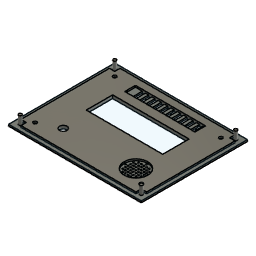
HousingLid v3 (Autodesk Fusion 360 design; units mm, degrees)
Autodesk Fusion 360 part; units mm, degrees
note: some values were not read from the file. Set by a fixed rule: which sketch regions a step uses; which face or edge a step refers to.
sketch "Sketch1" plane through (0, 0, 0) normal (0, 1, 0) x (1, 0, 0)
  line L0 (0, 0) -> (125, 0)
  line L1 (125, 0) -> (125, -100)
  line L2 (125, -100) -> (0, -100)
  line L3 (0, -100) -> (0, 0)
  dimension "d1" = 125
  dimension "d2" = 100
  constraint horizontal L0
  constraint vertical L1
  constraint horizontal L2
  constraint vertical L3
  constraint coincident L0.start L3.end
  measures "d1" distance of L0.start L0.end
  measures "d2" distance of L0.start L2.end
extrude "Extrude1" add sketch "Sketch1" along normal blind 2
sketch "Sketch2" plane through (0, 2, 0) normal (0, 1, 0) x (-1, 0, 0)
  line L0 (0, 100) -> (-125, 100)
  line L1 (-125, 100) -> (-125, 0)
  line L2 (-125, 0) -> (0, 0)
  line L3 (0, 0) -> (0, 100)
  line L4 (-10, 0) -> (-10, 3.3)
  line L5 (0, 3.3) -> (-3.3, 3.3)
  line L6 (-125, 100) -> (-121.7, 100)
  line L7 (-121.7, 100) -> (-121.7, 96.7)
  line L8 (-121.7, 96.7) -> (-125, 96.7)
  line L9 (-125, 96.7) -> (-125, 100)
  line L10 (-3.3, 3.3) -> (-121.7, 3.3)
  line L11 (-121.7, 3.3) -> (-121.7, 96.7)
  line L12 (-121.7, 96.7) -> (-3.3, 96.7)
  line L13 (-3.3, 96.7) -> (-3.3, 3.3)
  dimension "d5" = 3.3
  dimension "d6" = 3.3
  dimension "d7" = 3.3
  dimension "d8" = 3.3
  constraint coincident L2 L4.start
  constraint perpendicular L2 L4
  constraint coincident L3 L5.start
  constraint perpendicular L3 L5
  constraint horizontal L6
  constraint vertical L7
  constraint horizontal L8
  constraint vertical L9
  constraint coincident L0.end L1.start
  constraint horizontal L10
  constraint vertical L11
  constraint horizontal L12
  constraint vertical L13
  measures "d5" distance of L4.start L4.end
  measures "d6" distance of L5.start L5.end
  measures "d7" distance of L0.end L6.end
  measures "d8" distance of L0.end L8.end
extrude "Extrude2" add sketch "Sketch2" along normal blind 1 contours L10 L11 L12 L13
extrude "Extrude3" cut 1 faces at (42.7667, 2, 1.1) along direction (0, -1, 0) blind 0.5
sketch "Sketch3" plane through (0, 3, 0) normal (0, 1, 0) x (-1, 0, 0)
  line L0 (-3.3, 96.7) -> (-121.7, 96.7)
  line L1 (-121.7, 96.7) -> (-121.7, 3.3)
  line L2 (-121.7, 3.3) -> (-3.3, 3.3)
  line L3 (-3.3, 3.3) -> (-3.3, 96.7)
  line L4 (-3.3, 3.3) -> (-13.5, 3.3)
  line L5 (-13.5, 3.3) -> (-13.5, 13.5)
  line L6 (-13.5, 13.5) -> (-3.3, 13.5)
  line L7 (-3.3, 13.5) -> (-3.3, 3.3)
  line L8 (-3.3, 96.7) -> (-13.5, 96.7)
  line L9 (-13.5, 96.7) -> (-13.5, 86.5)
  line L10 (-13.5, 86.5) -> (-3.3, 86.5)
  line L11 (-3.3, 86.5) -> (-3.3, 96.7)
  line L12 (-121.7, 3.3) -> (-111.5, 3.3)
  line L13 (-111.5, 3.3) -> (-111.5, 13.5)
  line L14 (-111.5, 13.5) -> (-121.7, 13.5)
  line L15 (-121.7, 13.5) -> (-121.7, 3.3)
  line L16 (-121.7, 96.7) -> (-111.5, 96.7)
  line L17 (-111.5, 96.7) -> (-111.5, 86.5)
  line L18 (-111.5, 86.5) -> (-121.7, 86.5)
  line L19 (-121.7, 86.5) -> (-121.7, 96.7)
  dimension "d13" = 10.2
  dimension "d14" = 10.2
  dimension "d15" = 10.2
  dimension "d16" = 10.2
  dimension "d17" = 10.2
  dimension "d18" = 10.2
  dimension "d19" = 10.2
  dimension "d20" = 10.2
  constraint horizontal L4
  constraint vertical L5
  constraint horizontal L6
  constraint vertical L7
  constraint coincident L2.end L3.start
  constraint horizontal L8
  constraint vertical L9
  constraint horizontal L10
  constraint vertical L11
  constraint coincident L0.start L3.end
  constraint horizontal L12
  constraint vertical L13
  constraint horizontal L14
  constraint vertical L15
  constraint coincident L1.end L2.start
  constraint horizontal L16
  constraint vertical L17
  constraint horizontal L18
  constraint vertical L19
  constraint coincident L0.end L1.start
  measures "d13" distance of L2.end L4.end
  measures "d14" distance of L2.end L6.end
  measures "d15" distance of L0.start L8.end
  measures "d16" distance of L0.start L10.end
  measures "d17" distance of L1.end L12.end
  measures "d18" distance of L1.end L14.end
  measures "d19" distance of L0.end L16.end
  measures "d20" distance of L0.end L18.end
extrude "Extrude4" cut sketch "Sketch3" against normal blind 1 contours L0 L3 L8 L9 L10 L11 | L0 L1 L16 L17 L18 L19 | L2 L3 L4 L5 L6 L7 | L1 L2 L12 L13 L14 L15
extrude "Extrude5" cut 4 faces at (6.7, 2, 6.7) (118.3, 2, 6.7) (118.3, 2, 93.3) (6.7, 2, 93.3) along direction (0, -1, 0) blind 0.5
sketch "Sketch4" plane through (0, 1.5, 0) normal (0, 1, 0) x (-1, 0, 0)
  line L0 (-3.3, 13.5) -> (-13.5, 13.5)
  line L1 (-13.5, 13.5) -> (-13.5, 3.3)
  line L2 (-13.5, 3.3) -> (-111.5, 3.3)
  line L3 (-111.5, 3.3) -> (-111.5, 13.5)
  line L4 (-111.5, 13.5) -> (-121.7, 13.5)
  line L5 (-121.7, 13.5) -> (-121.7, 86.5)
  line L6 (-121.7, 86.5) -> (-111.5, 86.5)
  line L7 (-111.5, 86.5) -> (-111.5, 96.7)
  line L8 (-111.5, 96.7) -> (-13.5, 96.7)
  line L9 (-13.5, 96.7) -> (-13.5, 86.5)
  line L10 (-13.5, 86.5) -> (-3.3, 86.5)
  line L11 (-3.3, 86.5) -> (-3.3, 13.5)
  line L12 (0, 100) -> (-125, 100)
  line L13 (-125, 100) -> (-125, 0)
  line L14 (-125, 0) -> (0, 0)
  line L15 (0, 0) -> (0, 100)
  line L16 (0, 0) -> (-8, 0)
  line L17 (0, 8) -> (0, 0)
  circle A0 centre (-8, 8) radius 1.5
  line L18 (0, 100) -> (-8, 100)
  line L19 (-8, 100) -> (-8, 92)
  line L20 (-8, 92) -> (0, 92)
  line L21 (0, 92) -> (0, 100)
  circle A1 centre (-8, 92) radius 1.5
  line L22 (-125, 100) -> (-117, 100)
  line L23 (-117, 100) -> (-117, 92)
  line L24 (-117, 92) -> (-125, 92)
  line L25 (-125, 92) -> (-125, 100)
  circle A2 centre (-117, 92) radius 1.5
  line L26 (-125, 0) -> (-117, 0)
  line L27 (-117, 0) -> (-117, 8)
  line L28 (-117, 8) -> (-125, 8)
  line L29 (-125, 8) -> (-125, 0)
  circle A3 centre (-117, 8) radius 1.5
  dimension "d25" = 8
  dimension "d26" = 8
  dimension "d27" = 3
  dimension "d28" = 8
  dimension "d29" = 8
  dimension "d30" = 3
  dimension "d31" = 3
  dimension "d32" = 3
  constraint horizontal L16
  constraint vertical L17
  constraint coincident L14.end L15.start
  constraint horizontal L18
  constraint vertical L19
  constraint horizontal L20
  constraint vertical L21
  constraint coincident L12.start L15.end
  constraint coincident L19.end L20.start
  constraint horizontal L22
  constraint vertical L23
  constraint horizontal L24
  constraint vertical L25
  constraint coincident L12.end L13.start
  constraint coincident L23.end L24.start
  constraint horizontal L26
  constraint vertical L27
  constraint horizontal L28
  constraint vertical L29
  constraint coincident L13.end L14.start
  constraint coincident L27.end L28.start
  measures "d25" distance of L14.end L16.end
  measures "d26" distance of L14.end L17.start
  measures "d27" diameter of A0
  measures "d28" distance of L12.start L18.end
  measures "d29" distance of L12.start L20.end
  measures "d30" diameter of A1
  measures "d31" diameter of A2
  measures "d32" diameter of A3
extrude "Extrude6" add sketch "Sketch4" along normal blind 5 contours L19 L20 A1 | L19 L20 A1 | L23 L24 A2 | L23 L24 A2 | L27 L28 A3 | L27 L28 A3 | A0
extrude "Extrude7" add 4 faces at (8.1827, 6.5, 8.5095) (8.0374, 6.5, 90.9381) (117.5343, 6.5, 7.6091) (116.9626, 6.5, 92.2038) along direction (0, 1, 0) blind 8
extrude "Extrude8" cut 4 faces at (8.1827, 14.5, 8.5095) (8.0374, 14.5, 90.9381) (117.5343, 14.5, 7.6091) (116.9626, 14.5, 92.2038) along direction (0, -1, 0) blind 14.5
sketch "Sketch5" plane through (0, 1.5, 0) normal (0, 1, 0) x (-1, 0, 0)
  circle A0 centre (-8, 8) radius 1.5
  circle A1 centre (-117, 8) radius 1.5
  circle A2 centre (-8, 92) radius 1.5
  circle A3 centre (-117, 92) radius 1.5
  line L0 (-3.3, 13.5) -> (-13.5, 13.5)
  line L1 (-13.5, 13.5) -> (-13.5, 3.3)
  line L2 (-13.5, 3.3) -> (-111.5, 3.3)
  line L3 (-111.5, 3.3) -> (-111.5, 13.5)
  line L4 (-111.5, 13.5) -> (-121.7, 13.5)
  line L5 (-121.7, 13.5) -> (-121.7, 86.5)
  line L6 (-121.7, 86.5) -> (-111.5, 86.5)
  line L7 (-111.5, 86.5) -> (-111.5, 96.7)
  line L8 (-111.5, 96.7) -> (-13.5, 96.7)
  line L9 (-13.5, 96.7) -> (-13.5, 86.5)
  line L10 (-13.5, 86.5) -> (-3.3, 86.5)
  line L11 (-3.3, 86.5) -> (-3.3, 13.5)
  line L12 (0, 100) -> (-125, 100)
  line L13 (-125, 100) -> (-125, 0)
  line L14 (-125, 0) -> (0, 0)
  line L15 (0, 0) -> (0, 100)
  circle A4 centre (-8, 8) radius 1.65
  circle A5 centre (-8, 92) radius 1.65
  circle A6 centre (-117, 92) radius 1.65
  circle A7 centre (-117, 8) radius 1.65
  dimension "d39" = 3.3
  dimension "d40" = 3.3
  dimension "d41" = 3.3
  dimension "d42" = 3.3
  constraint concentric A0 A4
  constraint concentric A2 A5
  constraint concentric A3 A6
  constraint concentric A1 A7
  measures "d39" diameter of A4
  measures "d40" diameter of A5
  measures "d41" diameter of A6
  measures "d42" diameter of A7
extrude "Extrude9" cut sketch "Sketch5" against normal blind 1.5 contours A4 | A5 | A6 | A7
delete_face "DeleteFace1" 1 faces at (6.3521, 0.5, 7.9178)
delete_face "DeleteFace2" 1 faces at (9.4491, 0.5, 91.2109)
delete_face "DeleteFace3" 1 faces at (117.7527, 0.5, 93.4683)
delete_face "DeleteFace4" 1 faces at (117.7527, 0.5, 9.4683)
sketch "Sketch6" plane through (0, 0, 0) normal (0, -1, 0) x (1, 0, 0)
  line L0 (125, 100) -> (0, 100)
  line L1 (0, 100) -> (0, 0)
  line L2 (0, 0) -> (125, 0)
  line L3 (125, 0) -> (125, 100)
  line L4 (0, 0) -> (3, 0)
  line L5 (0, 3) -> (0, 0)
  line L6 (0, 100) -> (3, 100)
  line L7 (0, 97) -> (0, 100)
  line L8 (125, 100) -> (122, 100)
  line L9 (125, 97) -> (125, 100)
  line L10 (125, 0) -> (122, 0)
  line L11 (125, 3) -> (125, 0)
  circle A0 centre (122, 3) radius 1.65
  circle A1 centre (3, 3) radius 1.65
  circle A2 centre (3, 97) radius 1.65
  circle A3 centre (122, 97) radius 1.65
  dimension "d45" = 3
  dimension "d46" = 3
  dimension "d47" = 3
  dimension "d48" = 3
  dimension "d49" = 3
  dimension "d50" = 3.3
  dimension "d51" = 3.3
  dimension "d52" = 3.3
  dimension "d53" = 3.3
  constraint horizontal L4
  constraint vertical L5
  constraint coincident L1.end L2.start
  constraint horizontal L6
  constraint vertical L7
  constraint coincident L0.end L1.start
  constraint horizontal L8
  constraint vertical L9
  constraint coincident L0.start L3.end
  constraint horizontal L10
  constraint vertical L11
  constraint coincident L2.end L3.start
  measures "d45" distance of L0.end L7.start
  measures "d46" distance of L0.start L8.end
  measures "d47" distance of L0.start L9.start
  measures "d48" distance of L2.end L10.end
  measures "d49" distance of L2.end L11.start
  measures "d50" diameter of A0
  measures "d51" diameter of A1
  measures "d52" diameter of A2
  measures "d53" diameter of A3
extrude "Extrude10" cut sketch "Sketch6" against normal blind 1.5 contours A0 | A1 | A2 | A3
sketch "Sketch7" plane through (0, 1.5, 0) normal (0, 1, 0) x (-1, 0, 0)
  circle A0 centre (-3, 3) radius 1.65
  circle A1 centre (-122, 3) radius 1.65
  circle A2 centre (-3, 97) radius 1.65
  circle A3 centre (-122, 97) radius 1.65
  line L0 (-3.3, 13.5) -> (-13.5, 13.5)
  line L1 (-13.5, 13.5) -> (-13.5, 3.3)
  line L2 (-13.5, 3.3) -> (-111.5, 3.3)
  line L3 (-111.5, 3.3) -> (-111.5, 13.5)
  line L4 (-111.5, 13.5) -> (-121.7, 13.5)
  line L5 (-121.7, 13.5) -> (-121.7, 86.5)
  line L6 (-121.7, 86.5) -> (-111.5, 86.5)
  line L7 (-111.5, 86.5) -> (-111.5, 96.7)
  line L8 (-111.5, 96.7) -> (-13.5, 96.7)
  line L9 (-13.5, 96.7) -> (-13.5, 86.5)
  line L10 (-13.5, 86.5) -> (-3.3, 86.5)
  line L11 (-3.3, 86.5) -> (-3.3, 13.5)
  line L12 (0, 100) -> (-125, 100)
  line L13 (-125, 100) -> (-125, 0)
  line L14 (-125, 0) -> (0, 0)
  line L15 (0, 0) -> (0, 100)
  line L16 (0, 0) -> (-8.3, 0)
  line L17 (-8.3, 0) -> (-8.3, 8.3)
  line L18 (-8.3, 8.3) -> (0, 8.3)
  line L19 (0, 8.3) -> (0, 0)
  line L20 (-3.3, 13.5) -> (-3.3, 8.3)
  line L21 (-13.5, 3.3) -> (-8.3, 3.3)
  line L22 (-111.5, 3.3) -> (-116.7, 3.3)
  line L23 (-121.7, 13.5) -> (-121.7, 8.3)
  line L24 (-125, 0) -> (-116.7, 0)
  line L25 (-116.7, 0) -> (-116.7, 8.3)
  line L26 (-116.7, 8.3) -> (-125, 8.3)
  line L27 (-125, 8.3) -> (-125, 0)
  line L28 (-3.3, 86.5) -> (-13.5, 86.5)
  line L29 (-13.5, 86.5) -> (-13.5, 91.7)
  line L30 (-13.5, 91.7) -> (-3.3, 91.7)
  line L31 (-3.3, 91.7) -> (-3.3, 86.5)
  line L32 (-13.5, 96.7) -> (-8.3, 96.7)
  line L33 (-8.3, 96.7) -> (-8.3, 91.7)
  line L34 (-13.5, 91.7) -> (-13.5, 96.7)
  line L35 (-111.5, 96.7) -> (-116.7, 96.7)
  line L36 (-116.7, 96.7) -> (-116.7, 86.5)
  line L37 (-116.7, 86.5) -> (-111.5, 86.5)
  line L38 (-111.5, 86.5) -> (-111.5, 96.7)
  line L39 (-121.7, 86.5) -> (-111.5, 86.5)
  line L40 (-111.5, 86.5) -> (-111.5, 91.7)
  line L41 (-111.5, 91.7) -> (-121.7, 91.7)
  line L42 (-121.7, 91.7) -> (-121.7, 86.5)
  dimension "d59" = 8.3
  dimension "d60" = 8.3
  dimension "d61" = 5.2
  dimension "d62" = 5.2
  dimension "d63" = 8.3
  dimension "d64" = 8.3
  dimension "d65" = 5.2
  dimension "d66" = 5.2
  dimension "d67" = 5.2
  dimension "d68" = 5.2
  constraint horizontal L16
  constraint vertical L17
  constraint horizontal L18
  constraint vertical L19
  constraint coincident L14.end L15.start
  constraint coincident L0.start L11.end
  constraint coincident L18 L20.end
  constraint perpendicular L18 L20
  constraint coincident L1.end L2.start
  constraint coincident L17 L21.end
  constraint perpendicular L17 L21
  constraint coincident L2.end L3.start
  constraint perpendicular L3 L22
  constraint coincident L4.end L5.start
  constraint perpendicular L4 L23
  constraint horizontal L24
  constraint vertical L25
  constraint horizontal L26
  constraint vertical L27
  constraint coincident L13.end L14.start
  constraint horizontal L28
  constraint vertical L29
  constraint horizontal L30
  constraint vertical L31
  constraint coincident L10.end L11.start
  constraint horizontal L32
  constraint vertical L33
  constraint vertical L34
  constraint coincident L8.end L9.start
  constraint horizontal L35
  constraint vertical L36
  constraint horizontal L37
  constraint vertical L38
  constraint coincident L6 L36.end
  constraint coincident L7.end L8.start
  constraint horizontal L39
  constraint vertical L40
  constraint horizontal L41
  constraint vertical L42
  constraint coincident L5.end L6.start
  measures "d59" distance of L14.end L16.end
  measures "d60" distance of L14.end L18.end
  measures "d61" distance of L2.end L22.end
  measures "d62" distance of L4.end L23.end
  measures "d63" distance of L13.end L24.end
  measures "d64" distance of L13.end L26.end
  measures "d65" distance of L10.end L30.end
  measures "d66" distance of L8.end L32.end
  measures "d67" distance of L7.end L35.end
  measures "d68" distance of L5.end L41.end
extrude "Extrude11" add sketch "Sketch7" along normal blind 1.5 contours L0 L1 L17 L18 L20 L21 | L9 L10 L28 L29 L30 L31 | L3 L4 L22 L23 L25 L26 | L9 L30 L32 L33 L34 | L7 L35 L36 L38 L41 | L6 L36 L39 L41 L42 | L6 L7 L36 L37 L38 L39 L40 L41
delete_face "DeleteFace5" 1 faces at (121.2473, 1, 1.5317)
sketch "Sketch8" plane through (0, 1.5, 0) normal (0, 1, 0) x (-1, 0, 0)
  line L0 (-116.7, 96.7) -> (-8.3, 96.7)
  line L1 (-8.3, 96.7) -> (-8.3, 91.7)
  line L2 (-8.3, 91.7) -> (-3.3, 91.7)
  line L3 (-3.3, 91.7) -> (-3.3, 8.3)
  line L4 (-3.3, 8.3) -> (-8.3, 8.3)
  line L5 (-8.3, 8.3) -> (-8.3, 3.3)
  line L6 (-8.3, 3.3) -> (-116.7, 3.3)
  line L7 (-116.7, 3.3) -> (-116.7, 8.3)
  line L8 (-116.7, 8.3) -> (-121.7, 8.3)
  line L9 (-121.7, 8.3) -> (-121.7, 91.7)
  line L10 (-121.7, 91.7) -> (-116.7, 91.7)
  line L11 (-116.7, 91.7) -> (-116.7, 96.7)
  line L12 (0, 100) -> (-125, 100)
  line L13 (-125, 100) -> (-125, 0)
  line L14 (-125, 0) -> (0, 0)
  line L15 (0, 0) -> (0, 100)
delete_face "DeleteFace6" 1 faces at (4.4079, 1, 97.8604)
delete_face "DeleteFace7" 1 faces at (4.6479, 1, 2.9178)
delete_face "DeleteFace8" 1 faces at (122.4469, 1, 98.5883)
sketch "Sketch9" plane through (0, 1.5, 0) normal (0, 1, 0) x (-1, 0, 0)
  line L0 (0, 0) -> (-5.5, 0)
  line L1 (0, 5.5) -> (0, 0)
  line L2 (0, 100) -> (-5, 100)
  line L3 (0, 95) -> (0, 100)
  line L4 (-125, 100) -> (-119.5, 100)
  line L5 (-125, 94.5) -> (-125, 100)
  line L6 (0, 100) -> (-5.5, 100)
  line L7 (0, 94.5) -> (0, 100)
  line L8 (-125, 0) -> (-119.5, 0)
  line L9 (-125, 5.5) -> (-125, 0)
  circle A0 centre (-119.5, 5.5) radius 1.5
  circle A1 centre (-119.5, 94.5) radius 1.5
  circle A2 centre (-5.5, 94.5) radius 1.5
  circle A3 centre (-5.5, 5.5) radius 1.5
  dimension "d71" = 5.5
  dimension "d72" = 5.5
  dimension "d73" = 5.5
  dimension "d74" = 5.5
  dimension "d75" = 5.5
  dimension "d76" = 5.5
  dimension "d77" = 3
  dimension "d78" = 3
  dimension "d79" = 3
  dimension "d80" = 3
  constraint horizontal L0
  constraint vertical L1
  constraint coincident L0.start L1.end
  constraint horizontal L2
  constraint vertical L3
  constraint horizontal L4
  constraint vertical L5
  constraint horizontal L6
  constraint vertical L7
  constraint horizontal L8
  constraint vertical L9
  measures "d71" distance of L0.start L0.end
  measures "d72" distance of L0.start L1.start
  measures "d73" distance of L4.start L4.end
  measures "d74" distance of L4.start L5.start
  measures "d75" distance of L8.start L8.end
  measures "d76" distance of L8.start L9.start
  measures "d77" diameter of A0
  measures "d78" diameter of A1
  measures "d79" diameter of A2
  measures "d80" diameter of A3
extrude "Extrude12" add sketch "Sketch9" along normal blind 8
sketch "Sketch10" plane through (0, 3, 0) normal (0, 1, 0) x (-1, 0, 0)
  line L0 (-116.7, 3.3) -> (-8.3, 3.3)
  line L1 (-8.3, 3.3) -> (-8.3, 8.3)
  line L2 (-8.3, 8.3) -> (-3.3, 8.3)
  line L3 (-3.3, 8.3) -> (-3.3, 91.7)
  line L4 (-3.3, 91.7) -> (-8.3, 91.7)
  line L5 (-8.3, 91.7) -> (-8.3, 96.7)
  line L6 (-8.3, 96.7) -> (-116.7, 96.7)
  line L7 (-116.7, 96.7) -> (-116.7, 91.7)
  line L8 (-116.7, 91.7) -> (-121.7, 91.7)
  line L9 (-121.7, 91.7) -> (-121.7, 8.3)
  line L10 (-121.7, 8.3) -> (-116.7, 8.3)
  line L11 (-116.7, 8.3) -> (-116.7, 3.3)
  line L12 (-12.5, 12.5) -> (-12.5, 0)
  line L13 (0, 0) -> (-7.5, 0)
  line L14 (-7.5, 0) -> (-7.5, 7.5)
  line L15 (-7.5, 7.5) -> (-117.5, 7.5)
  line L16 (-117.5, 7.5) -> (-117.5, 92.5)
  line L17 (-117.5, 92.5) -> (-7.5, 92.5)
  line L18 (-7.5, 92.5) -> (-7.5, 7.5)
  line L19 (-26.5, 28.5) -> (-98.5, 28.5)
  line L20 (-98.5, 28.5) -> (-98.5, 53.3)
  line L21 (-98.5, 53.3) -> (-26.5, 53.3)
  line L22 (-26.5, 53.3) -> (-26.5, 28.5)
  line L23 (-117.5, 92.5) -> (-117.5, 79)
  line L24 (-117.5, 92.5) -> (-94.5, 92.5)
  line L25 (-117.5, 79) -> (-117.5, 92.5)
  circle A0 centre (-94.5, 79) radius 3.5
  line L26 (-7.5, 92.5) -> (-27.5, 92.5)
  line L27 (-7.5, 77.5) -> (-7.5, 92.5)
  circle A1 centre (-27.5, 77.5) radius 9
  line L28 (-7.5, 7.5) -> (-29.5, 7.5)
  line L29 (-29.5, 7.5) -> (-29.5, 10)
  line L30 (-29.5, 10) -> (-95.5, 10)
  line L31 (-95.5, 10) -> (-95.5, 20)
  line L32 (-95.5, 20) -> (-29.5, 20)
  line L33 (-29.5, 20) -> (-29.5, 10)
  line L34 (-33, 10) -> (-36, 10)
  line L35 (-36, 10) -> (-36, 20)
  line L36 (-36, 20) -> (-33, 20)
  line L37 (-33, 20) -> (-33, 10)
  line L38 (-39, 20) -> (-42, 20)
  line L39 (-42, 20) -> (-42, 10)
  line L40 (-42, 10) -> (-39, 10)
  line L41 (-39, 10) -> (-39, 20)
  line L42 (-45, 10) -> (-48, 10)
  line L43 (-48, 10) -> (-48, 20)
  line L44 (-48, 20) -> (-45, 20)
  line L45 (-45, 20) -> (-45, 10)
  line L46 (-51, 20) -> (-54, 20)
  line L47 (-54, 20) -> (-54, 10)
  line L48 (-54, 10) -> (-51, 10)
  line L49 (-51, 10) -> (-51, 20)
  line L50 (-57, 10) -> (-60, 10)
  line L51 (-60, 10) -> (-60, 20)
  line L52 (-60, 20) -> (-57, 20)
  line L53 (-57, 20) -> (-57, 10)
  line L54 (-63, 20) -> (-66, 20)
  line L55 (-66, 20) -> (-66, 10)
  line L56 (-66, 10) -> (-63, 10)
  line L57 (-63, 10) -> (-63, 20)
  line L58 (-69, 10) -> (-72, 10)
  line L59 (-72, 10) -> (-72, 20)
  line L60 (-72, 20) -> (-69, 20)
  line L61 (-69, 20) -> (-69, 10)
  line L62 (-75, 10) -> (-78, 10)
  line L63 (-78, 10) -> (-78, 20)
  line L64 (-78, 20) -> (-75, 20)
  line L65 (-75, 20) -> (-75, 10)
  line L66 (-81, 10) -> (-84, 10)
  line L67 (-84, 10) -> (-84, 20)
  line L68 (-84, 20) -> (-81, 20)
  line L69 (-81, 20) -> (-81, 10)
  line L70 (-87, 10) -> (-90, 10)
  line L71 (-90, 10) -> (-90, 20)
  line L72 (-90, 20) -> (-87, 20)
  line L73 (-87, 20) -> (-87, 10)
  line L74 (-93, 10) -> (-95.5, 10)
  line L75 (-95.5, 10) -> (-95.5, 20)
  line L76 (-95.5, 20) -> (-93, 20)
  line L77 (-93, 20) -> (-93, 10)
  dimension "d85" = 7.5
  dimension "d86" = 7.5
  dimension "d87" = 110
  dimension "d88" = 85
  dimension "d92" = 24.8
  dimension "d93" = 23
  dimension "d94" = 13.5
  dimension "d95" = 7
  dimension "d96" = 20
  dimension "d97" = 15
  dimension "d98" = 18
  dimension "d99" = 22
  dimension "d100" = 66
  dimension "d101" = 10
  constraint coincident L13.start origin
  constraint horizontal L13
  constraint perpendicular L13 L14
  constraint horizontal L15
  constraint vertical L16
  constraint horizontal L17
  constraint vertical L18
  constraint horizontal L19
  constraint vertical L20
  constraint horizontal L21
  constraint vertical L22
  constraint coincident L16 L23.end
  constraint horizontal L24
  constraint vertical L25
  constraint horizontal L26
  constraint vertical L27
  constraint perpendicular L1 L28
  constraint perpendicular L15 L29
  constraint horizontal L30
  constraint vertical L31
  constraint horizontal L32
  constraint vertical L33
  constraint horizontal L34
  constraint vertical L35
  constraint horizontal L36
  constraint vertical L37
  constraint coincident L32 L35.end
  constraint coincident L30 L34.start
  constraint horizontal L38
  constraint vertical L39
  constraint horizontal L40
  constraint vertical L41
  constraint coincident L30 L39.end
  constraint coincident L32 L38.start
  constraint horizontal L42
  constraint vertical L43
  constraint horizontal L44
  constraint vertical L45
  constraint coincident L32 L43.end
  constraint coincident L30 L42.start
  constraint horizontal L46
  constraint vertical L47
  constraint horizontal L48
  constraint vertical L49
  constraint coincident L30 L47.end
  constraint coincident L32 L46.start
  constraint horizontal L50
  constraint vertical L51
  constraint horizontal L52
  constraint vertical L53
  constraint coincident L32 L51.end
  constraint coincident L30 L50.start
  constraint horizontal L54
  constraint vertical L55
  constraint horizontal L56
  constraint vertical L57
  constraint coincident L30 L55.end
  constraint coincident L32 L54.start
  constraint horizontal L58
  constraint vertical L59
  constraint horizontal L60
  constraint vertical L61
  constraint coincident L32 L59.end
  constraint coincident L30 L58.start
  constraint horizontal L62
  constraint vertical L63
  constraint horizontal L64
  constraint vertical L65
  constraint coincident L32 L63.end
  constraint coincident L30 L62.start
  constraint horizontal L66
  constraint vertical L67
  constraint horizontal L68
  constraint vertical L69
  constraint coincident L32 L67.end
  constraint coincident L30 L66.start
  constraint horizontal L70
  constraint vertical L71
  constraint horizontal L72
  constraint vertical L73
  constraint coincident L32 L71.end
  constraint coincident L30 L70.start
  constraint horizontal L74
  constraint vertical L75
  constraint horizontal L76
  constraint vertical L77
  constraint coincident L30 L74.start
  measures "d85" distance of L13.start L13.end
  measures "d86" distance of L13.end L14.end
  measures "d87" distance of L14.end L15.end
  measures "d88" distance of L14.end L17.end
  measures "d92" distance of L19.start L21.end
  measures "d93" distance of L16.end L24.end
  measures "d94" distance of L16.end L23.end
  measures "d95" diameter of A0
  measures "d96" distance of L17.end L26.end
  measures "d97" distance of L17.end L27.start
  measures "d98" diameter of A1
  measures "d99" distance of L14.end L28.end
  measures "d100" distance of L29.end L30.end
  measures "d101" distance of L29.end L32.end
extrude "Extrude13" cut sketch "Sketch10" against normal blind 3 contours L19 L20 L21 L22 | A0 | L30 L32 L35 L41 | L30 L32 L39 L45 | L30 L32 L43 L49 | L30 L32 L47 L53 | L30 L32 L51 L57 | L30 L32 L55 L61 | L30 L32 L59 L65 | L30 L32 L63 L69 | L30 L32 L67 L73 | L30 L32 L71 L77
delete_face "DeleteFace9" 1 faces at (91.0044, 1, 78.8255)
sketch "Sketch11" plane through (0, 3, 0) normal (0, 1, 0) x (-1, 0, 0)
  line L0 (-87, 20) -> (-84, 20)
  line L1 (-84, 20) -> (-84, 10)
  line L2 (-84, 10) -> (-87, 10)
  line L3 (-87, 10) -> (-87, 20)
  line L4 (-63, 20) -> (-60, 20)
  line L5 (-60, 20) -> (-60, 10)
  line L6 (-60, 10) -> (-63, 10)
  line L7 (-63, 10) -> (-63, 20)
  line L8 (-39, 20) -> (-36, 20)
  line L9 (-36, 20) -> (-36, 10)
  line L10 (-36, 10) -> (-39, 10)
  line L11 (-39, 10) -> (-39, 20)
  line L12 (-45, 10) -> (-45, 20)
  line L13 (-45, 20) -> (-42, 20)
  line L14 (-42, 20) -> (-42, 10)
  line L15 (-42, 10) -> (-45, 10)
  line L16 (-69, 10) -> (-69, 20)
  line L17 (-69, 20) -> (-66, 20)
  line L18 (-66, 20) -> (-66, 10)
  line L19 (-66, 10) -> (-69, 10)
  line L20 (-93, 20) -> (-90, 20)
  line L21 (-90, 20) -> (-90, 10)
  line L22 (-90, 10) -> (-93, 10)
  line L23 (-93, 10) -> (-93, 20)
  line L24 (-81, 20) -> (-78, 20)
  line L25 (-78, 20) -> (-78, 10)
  line L26 (-78, 10) -> (-81, 10)
  line L27 (-81, 10) -> (-81, 20)
  line L28 (-57, 10) -> (-57, 20)
  line L29 (-57, 20) -> (-54, 20)
  line L30 (-54, 20) -> (-54, 10)
  line L31 (-54, 10) -> (-57, 10)
  line L32 (-98.5, 28.5) -> (-98.5, 53.3)
  line L33 (-98.5, 53.3) -> (-26.5, 53.3)
  line L34 (-26.5, 53.3) -> (-26.5, 28.5)
  line L35 (-26.5, 28.5) -> (-98.5, 28.5)
  line L36 (-51, 20) -> (-48, 20)
  line L37 (-48, 20) -> (-48, 10)
  line L38 (-48, 10) -> (-51, 10)
  line L39 (-51, 10) -> (-51, 20)
  line L40 (-75, 20) -> (-72, 20)
  line L41 (-72, 20) -> (-72, 10)
  line L42 (-72, 10) -> (-75, 10)
  line L43 (-75, 10) -> (-75, 20)
  line L44 (-116.7, 3.3) -> (-8.3, 3.3)
  line L45 (-8.3, 3.3) -> (-8.3, 8.3)
  line L46 (-8.3, 8.3) -> (-3.3, 8.3)
  line L47 (-3.3, 8.3) -> (-3.3, 91.7)
  line L48 (-3.3, 91.7) -> (-8.3, 91.7)
  line L49 (-8.3, 91.7) -> (-8.3, 96.7)
  line L50 (-8.3, 96.7) -> (-116.7, 96.7)
  line L51 (-116.7, 96.7) -> (-116.7, 91.7)
  line L52 (-116.7, 91.7) -> (-121.7, 91.7)
  line L53 (-121.7, 91.7) -> (-121.7, 8.3)
  line L54 (-121.7, 8.3) -> (-116.7, 8.3)
  line L55 (-116.7, 8.3) -> (-116.7, 3.3)
  line L56 (-37.5, 10) -> (-37.5, 7.5)
  line L57 (-37.5, 7.5) -> (0, 7.5)
  line L58 (0, 0) -> (-7.5, 0)
  line L59 (-7.5, 0) -> (-7.5, 7.5)
  line L60 (-7.5, 7.5) -> (0, 7.5)
  line L61 (0, 7.5) -> (0, 0)
  line L62 (-125, 100) -> (-117.5, 100)
  line L63 (-117.5, 100) -> (-117.5, 92.5)
  line L64 (-117.5, 92.5) -> (-125, 92.5)
  line L65 (-125, 92.5) -> (-125, 100)
  line L66 (-7.5, 7.5) -> (-117.5, 7.5)
  line L67 (-117.5, 7.5) -> (-117.5, 92.5)
  line L68 (-117.5, 92.5) -> (-7.5, 92.5)
  line L69 (-7.5, 92.5) -> (-7.5, 7.5)
  line L70 (-117.5, 7.5) -> (-95.5, 7.5)
  line L71 (-95.5, 7.5) -> (-95.5, 10)
  line L72 (-7.5, 7.5) -> (-29.5, 7.5)
  line L73 (-29.5, 7.5) -> (-29.5, 10)
  line L74 (-29.5, 10) -> (-95.5, 10)
  line L75 (-95.5, 10) -> (-95.5, 20)
  line L76 (-95.5, 20) -> (-29.5, 20)
  line L77 (-29.5, 20) -> (-29.5, 10)
  line L78 (-117.5, 92.5) -> (-97.5, 92.5)
  line L79 (-97.5, 92.5) -> (-97.5, 77.5)
  line L80 (-97.5, 77.5) -> (-117.5, 77.5)
  line L81 (-117.5, 77.5) -> (-117.5, 92.5)
  circle A0 centre (-97.5, 77.5) radius 11.1
  dimension "d104" = 2.5
  dimension "d105" = 7.5
  dimension "d106" = 7.5
  dimension "d107" = 7.5
  dimension "d108" = 22
  dimension "d109" = 22
  dimension "d110" = 20
  dimension "d111" = 15
  dimension "d112" = 22.2
  constraint midpoint L10 L56.start
  constraint perpendicular L44 L56
  constraint perpendicular L47 L57
  constraint horizontal L58
  constraint vertical L59
  constraint horizontal L60
  constraint vertical L61
  constraint coincident L58.start L61.end
  constraint horizontal L62
  constraint vertical L63
  constraint horizontal L64
  constraint vertical L65
  constraint horizontal L66
  constraint vertical L67
  constraint horizontal L68
  constraint vertical L69
  constraint perpendicular L55 L70
  constraint perpendicular L70 L71
  constraint perpendicular L59 L72
  constraint perpendicular L72 L73
  constraint horizontal L74
  constraint vertical L75
  constraint horizontal L76
  constraint vertical L77
  constraint horizontal L78
  constraint vertical L79
  constraint horizontal L80
  constraint vertical L81
  constraint coincident L79.end L80.start
  measures "d104" distance of L56.start L56.end
  measures "d105" distance of L58.start L58.end
  measures "d106" distance of L62.start L62.end
  measures "d107" distance of L62.start L64.end
  measures "d108" distance of L66.end L70.end
  measures "d109" distance of L59.end L72.end
  measures "d110" distance of L63.end L78.end
  measures "d111" distance of L63.end L80.end
  measures "d112" diameter of A0
extrude "Extrude14" cut sketch "Sketch11" against normal blind 1.5 contours L3 L21 L74 L76 | L1 L27 L74 L76 | L23 L74 L75 L76 | L25 L43 L74 L76 | L16 L41 L74 L76 | L7 L18 L74 L76 | L9 L74 L76 L77 | L11 L14 L74 L76 | L5 L28 L74 L76 | L12 L37 L74 L76 | L79 L80 A0 | L79 L80 A0 | L30 L39 L74 L76
sketch "Sketch12" plane through (0, 3, 0) normal (0, 1, 0) x (-1, 0, 0)
  line L0 (-116.7, 3.3) -> (-8.3, 3.3)
  line L1 (-8.3, 3.3) -> (-8.3, 8.3)
  line L2 (-8.3, 8.3) -> (-3.3, 8.3)
  line L3 (-3.3, 8.3) -> (-3.3, 91.7)
  line L4 (-3.3, 91.7) -> (-8.3, 91.7)
  line L5 (-8.3, 91.7) -> (-8.3, 96.7)
  line L6 (-8.3, 96.7) -> (-116.7, 96.7)
  line L7 (-116.7, 96.7) -> (-116.7, 91.7)
  line L8 (-116.7, 91.7) -> (-121.7, 91.7)
  line L9 (-121.7, 91.7) -> (-121.7, 8.3)
  line L10 (-121.7, 8.3) -> (-116.7, 8.3)
  line L11 (-116.7, 8.3) -> (-116.7, 3.3)
  line L12 (-98.5, 28.5) -> (-98.5, 53.3)
  line L13 (-98.5, 53.3) -> (-26.5, 53.3)
  line L14 (-26.5, 53.3) -> (-26.5, 28.5)
  line L15 (-26.5, 28.5) -> (-98.5, 28.5)
  circle A0 centre (-97.5, 77.5) radius 11.1
  line L16 (-95.5, 20) -> (-29.5, 20)
  line L17 (-29.5, 20) -> (-29.5, 10)
  line L18 (-29.5, 10) -> (-95.5, 10)
  line L19 (-95.5, 10) -> (-95.5, 20)
  line L20 (0, 100) -> (-7.5, 100)
  line L21 (-7.5, 100) -> (-7.5, 92.5)
  line L22 (-7.5, 92.5) -> (0, 92.5)
  line L23 (0, 92.5) -> (0, 100)
  line L24 (-125, 0) -> (-117.5, 0)
  line L25 (-117.5, 0) -> (-117.5, 7.5)
  line L26 (-117.5, 7.5) -> (-125, 7.5)
  line L27 (-125, 7.5) -> (-125, 0)
  line L28 (-7.5, 92.5) -> (-117.5, 92.5)
  line L29 (-117.5, 92.5) -> (-117.5, 7.5)
  line L30 (-117.5, 7.5) -> (-7.5, 7.5)
  line L31 (-7.5, 7.5) -> (-7.5, 92.5)
  line L32 (-7.5, 92.5) -> (-30.5, 92.5)
  line L33 (-7.5, 79) -> (-7.5, 92.5)
  circle A1 centre (-30.5, 79) radius 3.5
  dimension "d115" = 7.5
  dimension "d116" = 7.5
  dimension "d117" = 7.5
  dimension "d118" = 7.5
  dimension "d119" = 23
  dimension "d120" = 13.5
  dimension "d121" = 7
  constraint horizontal L20
  constraint vertical L21
  constraint horizontal L22
  constraint vertical L23
  constraint horizontal L24
  constraint vertical L25
  constraint horizontal L26
  constraint vertical L27
  constraint horizontal L28
  constraint vertical L29
  constraint horizontal L30
  constraint vertical L31
  constraint horizontal L32
  constraint vertical L33
  measures "d115" distance of L20.start L20.end
  measures "d116" distance of L20.start L22.end
  measures "d117" distance of L24.start L24.end
  measures "d118" distance of L24.start L26.end
  measures "d119" distance of L21.end L32.end
  measures "d120" distance of L21.end L33.start
  measures "d121" diameter of A1
extrude "Extrude15" cut sketch "Sketch12" against normal blind 3 contours A1
sketch "Sketch13" plane through (0, 3, 0) normal (0, 1, 0) x (-1, 0, 0)
  circle A0 centre (-30.5, 79) radius 3.5
  line L0 (-116.7, 3.3) -> (-8.3, 3.3)
  line L1 (-8.3, 3.3) -> (-8.3, 8.3)
  line L2 (-8.3, 8.3) -> (-3.3, 8.3)
  line L3 (-3.3, 8.3) -> (-3.3, 91.7)
  line L4 (-3.3, 91.7) -> (-8.3, 91.7)
  line L5 (-8.3, 91.7) -> (-8.3, 96.7)
  line L6 (-8.3, 96.7) -> (-116.7, 96.7)
  line L7 (-116.7, 96.7) -> (-116.7, 91.7)
  line L8 (-116.7, 91.7) -> (-121.7, 91.7)
  line L9 (-121.7, 91.7) -> (-121.7, 8.3)
  line L10 (-121.7, 8.3) -> (-116.7, 8.3)
  line L11 (-116.7, 8.3) -> (-116.7, 3.3)
  line L12 (-98.5, 28.5) -> (-98.5, 53.3)
  line L13 (-98.5, 53.3) -> (-26.5, 53.3)
  line L14 (-26.5, 53.3) -> (-26.5, 28.5)
  line L15 (-26.5, 28.5) -> (-98.5, 28.5)
  circle A1 centre (-97.5, 77.5) radius 11.1
  line L16 (-95.5, 20) -> (-29.5, 20)
  line L17 (-29.5, 20) -> (-29.5, 10)
  line L18 (-29.5, 10) -> (-95.5, 10)
  line L19 (-95.5, 10) -> (-95.5, 20)
  line L20 (0, 0) -> (-7.5, 0)
  line L21 (-7.5, 0) -> (-7.5, 7.5)
  line L22 (-7.5, 7.5) -> (0, 7.5)
  line L23 (0, 7.5) -> (0, 0)
  line L24 (-125, 100) -> (-117.5, 100)
  line L25 (-117.5, 100) -> (-117.5, 92.5)
  line L26 (-117.5, 92.5) -> (-125, 92.5)
  line L27 (-125, 92.5) -> (-125, 100)
  line L28 (-117.5, 92.5) -> (-7.5, 92.5)
  line L29 (-7.5, 92.5) -> (-7.5, 7.5)
  line L30 (-7.5, 7.5) -> (-117.5, 7.5)
  line L31 (-117.5, 7.5) -> (-117.5, 92.5)
  line L32 (-7.5, 7.5) -> (-12.5, 7.5)
  line L33 (-7.5, 12.5) -> (-7.5, 7.5)
  line L34 (-7.5, 92.5) -> (-12.5, 92.5)
  line L35 (-7.5, 87.5) -> (-7.5, 92.5)
  line L36 (-117.5, 92.5) -> (-112.5, 92.5)
  line L37 (-117.5, 87.5) -> (-117.5, 92.5)
  line L38 (-117.5, 7.5) -> (-112.5, 7.5)
  line L39 (-117.5, 12.5) -> (-117.5, 7.5)
  circle A2 centre (-112.5, 12.5) radius 1.65
  circle A3 centre (-12.5, 12.5) radius 1.65
  circle A4 centre (-12.5, 87.5) radius 1.65
  circle A5 centre (-112.5, 87.5) radius 1.65
  dimension "d124" = 7.5
  dimension "d125" = 7.5
  dimension "d126" = 7.5
  dimension "d127" = 7.5
  dimension "d128" = 5
  dimension "d129" = 5
  dimension "d130" = 5
  dimension "d131" = 5
  dimension "d132" = 5
  dimension "d133" = 5
  dimension "d134" = 5
  dimension "d135" = 5
  dimension "d136" = 3.3
  dimension "d137" = 3.3
  dimension "d138" = 3.3
  dimension "d139" = 3.3
  constraint horizontal L20
  constraint vertical L21
  constraint horizontal L22
  constraint vertical L23
  constraint coincident L20.start L23.end
  constraint horizontal L24
  constraint vertical L25
  constraint horizontal L26
  constraint vertical L27
  constraint horizontal L28
  constraint vertical L29
  constraint horizontal L30
  constraint vertical L31
  constraint horizontal L32
  constraint vertical L33
  constraint horizontal L34
  constraint vertical L35
  constraint horizontal L36
  constraint vertical L37
  constraint horizontal L38
  constraint vertical L39
  measures "d124" distance of L20.start L20.end
  measures "d125" distance of L20.start L22.end
  measures "d126" distance of L24.start L24.end
  measures "d127" distance of L24.start L26.end
  measures "d128" distance of L21.end L32.end
  measures "d129" distance of L21.end L33.start
  measures "d130" distance of L28.end L34.end
  measures "d131" distance of L28.end L35.start
  measures "d132" distance of L25.end L36.end
  measures "d133" distance of L25.end L37.start
  measures "d134" distance of L30.end L38.end
  measures "d135" distance of L30.end L39.start
  measures "d136" diameter of A2
  measures "d137" diameter of A3
  measures "d138" diameter of A4
  measures "d139" diameter of A5
extrude "Extrude16" cut sketch "Sketch13" against normal blind 3 contours A2 | A3 | A4 | A5
sketch "Sketch14" plane through (0, 0, 0) normal (0, -1, 0) x (1, 0, 0)
  circle A0 centre (12.5, 87.5) radius 1.65
  circle A1 centre (112.5, 12.5) radius 1.65
  circle A2 centre (12.5, 12.5) radius 1.65
  circle A3 centre (112.5, 87.5) radius 1.65
  circle A4 centre (30.5, 79) radius 3.5
  line L0 (84, 20) -> (87, 20)
  line L1 (87, 20) -> (87, 10)
  line L2 (87, 10) -> (84, 10)
  line L3 (84, 10) -> (84, 20)
  line L4 (60, 20) -> (63, 20)
  line L5 (63, 20) -> (63, 10)
  line L6 (63, 10) -> (60, 10)
  line L7 (60, 10) -> (60, 20)
  line L8 (36, 20) -> (39, 20)
  line L9 (39, 20) -> (39, 10)
  line L10 (39, 10) -> (36, 10)
  line L11 (36, 10) -> (36, 20)
  line L12 (45, 20) -> (45, 10)
  line L13 (45, 10) -> (42, 10)
  line L14 (42, 10) -> (42, 20)
  line L15 (42, 20) -> (45, 20)
  line L16 (69, 20) -> (69, 10)
  line L17 (69, 10) -> (66, 10)
  line L18 (66, 10) -> (66, 20)
  line L19 (66, 20) -> (69, 20)
  line L20 (90, 20) -> (93, 20)
  line L21 (93, 20) -> (93, 10)
  line L22 (93, 10) -> (90, 10)
  line L23 (90, 10) -> (90, 20)
  line L24 (78, 20) -> (81, 20)
  line L25 (81, 20) -> (81, 10)
  line L26 (81, 10) -> (78, 10)
  line L27 (78, 10) -> (78, 20)
  line L28 (57, 20) -> (57, 10)
  line L29 (57, 10) -> (54, 10)
  line L30 (54, 10) -> (54, 20)
  line L31 (54, 20) -> (57, 20)
  line L32 (98.5, 53.3) -> (98.5, 28.5)
  line L33 (98.5, 28.5) -> (26.5, 28.5)
  line L34 (26.5, 28.5) -> (26.5, 53.3)
  line L35 (26.5, 53.3) -> (98.5, 53.3)
  line L36 (48, 20) -> (51, 20)
  line L37 (51, 20) -> (51, 10)
  line L38 (51, 10) -> (48, 10)
  line L39 (48, 10) -> (48, 20)
  line L40 (72, 20) -> (75, 20)
  line L41 (75, 20) -> (75, 10)
  line L42 (75, 10) -> (72, 10)
  line L43 (72, 10) -> (72, 20)
  line L44 (125, 100) -> (0, 100)
  line L45 (0, 100) -> (0, 0)
  line L46 (0, 0) -> (125, 0)
  line L47 (125, 0) -> (125, 100)
  circle A5 centre (12.5, 12.5) radius 3.5
  circle A6 centre (12.5, 87.5) radius 3.5
  circle A7 centre (112.5, 87.5) radius 3.5
  circle A8 centre (112.5, 12.5) radius 3.5
  dimension "d142" = 7
  dimension "d143" = 7
  dimension "d144" = 7
  dimension "d145" = 7
  constraint concentric A2 A5
  constraint concentric A0 A6
  constraint concentric A3 A7
  constraint concentric A1 A8
  measures "d142" diameter of A5
  measures "d143" diameter of A6
  measures "d144" diameter of A7
  measures "d145" diameter of A8
extrude "Extrude17" cut sketch "Sketch14" against normal blind 1 contours A5 | A6 | A7 | A8
extrude "Extrude18" cut 4 faces at (14.9695, 1, 86.0268) (110.0305, 1, 86.0268) (115.3642, 1, 12.2441) (15.3703, 1, 12.3261) along direction (0, 1, 0) blind 0.5
sketch "Sketch15" plane through (0, 1.5, 0) normal (0, 1, 0) x (-1, 0, 0)
  circle A0 centre (-95, 75) radius 0.75
  circle A1 centre (-97.5, 75) radius 0.75
  circle A2 centre (-100, 75) radius 0.75
  circle A3 centre (-102.5, 75) radius 0.75
  circle A4 centre (-95, 77.5) radius 0.75
  circle A5 centre (-97.5, 77.5) radius 0.75
  circle A6 centre (-100, 77.5) radius 0.75
  circle A7 centre (-102.5, 77.5) radius 0.75
  circle A8 centre (-105, 77.5) radius 0.75
  circle A9 centre (-105, 75) radius 0.75
  circle A10 centre (-92.5, 75) radius 0.75
  circle A11 centre (-92.5, 77.5) radius 0.75
  circle A12 centre (-90, 75) radius 0.75
  circle A13 centre (-90, 77.5) radius 0.75
  circle A14 centre (-87.5, 77.5) radius 0.75
  circle A15 centre (-107.5, 77.5) radius 0.75
  circle A16 centre (-105, 80) radius 0.75
  circle A17 centre (-102.5, 80) radius 0.75
  circle A18 centre (-100, 80) radius 0.75
  circle A19 centre (-97.5, 80) radius 0.75
  circle A20 centre (-95, 80) radius 0.75
  circle A21 centre (-92.5, 80) radius 0.75
  circle A22 centre (-90, 80) radius 0.75
  circle A23 centre (-97.5, 82.5) radius 0.75
  circle A24 centre (-95, 82.5) radius 0.75
  circle A25 centre (-92.5, 82.5) radius 0.75
  circle A26 centre (-97.5, 85) radius 0.75
  circle A27 centre (-95, 85) radius 0.75
  circle A28 centre (-97.5, 87.5) radius 0.75
  circle A29 centre (-100, 85) radius 0.75
  circle A30 centre (-100, 82.5) radius 0.75
  circle A31 centre (-102.5, 82.5) radius 0.75
  circle A32 centre (-97.5, 72.5) radius 0.75
  circle A33 centre (-97.5, 70) radius 0.75
  circle A34 centre (-97.5, 67.5) radius 0.75
  circle A35 centre (-95, 72.5) radius 0.75
  circle A36 centre (-92.5, 72.5) radius 0.75
  circle A37 centre (-95, 70) radius 0.75
  circle A38 centre (-92.5, 70) radius 0.75
  circle A39 centre (-90, 72.5) radius 0.75
  circle A40 centre (-90, 82.5) radius 0.75
  circle A41 centre (-92.5, 85) radius 0.75
  circle A42 centre (-102.5, 85) radius 0.75
  circle A43 centre (-105, 82.5) radius 0.75
  circle A44 centre (-100, 70) radius 0.75
  circle A45 centre (-100, 72.5) radius 0.75
  circle A46 centre (-102.5, 72.5) radius 0.75
  circle A47 centre (-102.5, 70) radius 0.75
  circle A48 centre (-105, 72.5) radius 0.75
  dimension "d150" = 1.5
  dimension "d151" = 1.5
  dimension "d152" = 1.5
  dimension "d153" = 1.5
  dimension "d154" = 1.5
  dimension "d155" = 1.5
  dimension "d156" = 1.5
  dimension "d157" = 1.5
  dimension "d158" = 1.5
  dimension "d159" = 1.5
  dimension "d160" = 1.5
  dimension "d161" = 1.5
  dimension "d162" = 1.5
  dimension "d163" = 1.5
  dimension "d164" = 1.5
  dimension "d165" = 1.5
  dimension "d166" = 1.5
  dimension "d167" = 1.5
  dimension "d168" = 1.5
  dimension "d169" = 1.5
  dimension "d170" = 1.5
  dimension "d171" = 1.5
  dimension "d172" = 1.5
  dimension "d173" = 1.5
  dimension "d174" = 1.5
  dimension "d175" = 1.5
  dimension "d176" = 1.5
  dimension "d177" = 1.5
  dimension "d178" = 1.5
  dimension "d179" = 1.5
  dimension "d180" = 1.5
  dimension "d181" = 1.5
  dimension "d182" = 1.5
  dimension "d183" = 1.5
  dimension "d184" = 1.5
  dimension "d185" = 1.5
  dimension "d186" = 1.5
  dimension "d187" = 1.5
  dimension "d188" = 1.5
  dimension "d189" = 1.5
  dimension "d190" = 1.5
  dimension "d191" = 1.5
  dimension "d192" = 1.5
  dimension "d193" = 1.5
  dimension "d194" = 1.5
  dimension "d195" = 1.5
  dimension "d196" = 1.5
  dimension "d197" = 1.5
  dimension "d198" = 1.5
  measures "d150" diameter of A0
  measures "d151" diameter of A1
  measures "d152" diameter of A2
  measures "d153" diameter of A3
  measures "d154" diameter of A4
  measures "d155" diameter of A5
  measures "d156" diameter of A6
  measures "d157" diameter of A7
  measures "d158" diameter of A8
  measures "d159" diameter of A9
  measures "d160" diameter of A10
  measures "d161" diameter of A11
  measures "d162" diameter of A12
  measures "d163" diameter of A13
  measures "d164" diameter of A14
  measures "d165" diameter of A15
  measures "d166" diameter of A16
  measures "d167" diameter of A17
  measures "d168" diameter of A18
  measures "d169" diameter of A19
  measures "d170" diameter of A20
  measures "d171" diameter of A21
  measures "d172" diameter of A22
  measures "d173" diameter of A23
  measures "d174" diameter of A24
  measures "d175" diameter of A25
  measures "d176" diameter of A26
  measures "d177" diameter of A27
  measures "d178" diameter of A28
  measures "d179" diameter of A29
  measures "d180" diameter of A30
  measures "d181" diameter of A31
  measures "d182" diameter of A32
  measures "d183" diameter of A33
  measures "d184" diameter of A34
  measures "d185" diameter of A35
  measures "d186" diameter of A36
  measures "d187" diameter of A37
  measures "d188" diameter of A38
  measures "d189" diameter of A39
  measures "d190" diameter of A40
  measures "d191" diameter of A41
  measures "d192" diameter of A42
  measures "d193" diameter of A43
  measures "d194" diameter of A44
  measures "d195" diameter of A45
  measures "d196" diameter of A46
  measures "d197" diameter of A47
  measures "d198" diameter of A48
extrude "Extrude19" cut sketch "Sketch15" against normal blind 1.5
